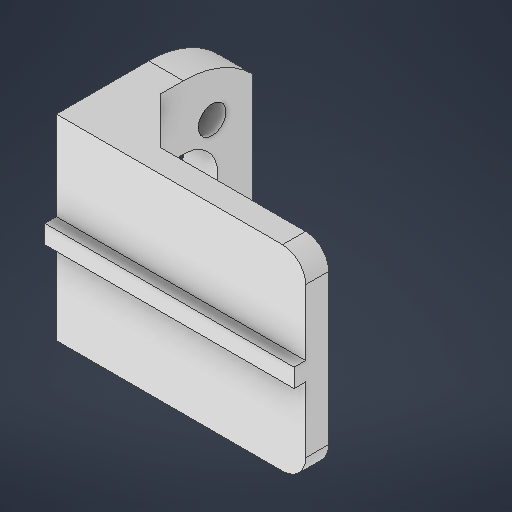
# Autodesk Inventor part: Trzymak2
Saved by Autodesk Inventor 2026 (Build 300175000, 175)
## iProperties
Created: 2025-04-24
Part Number: Trzymak2
Material: Generic
Document SubType Name: Modeling
Designer: isan
Density: 1 g/cm^3
Appearance: Default
Author: isan
Autodesk Inventor part; units mm, degrees
ref_plane "YZ Plane" through (0, 0, 0) normal (1, 0, 0) x (0, 1, 0)
ref_plane "XZ Plane" through (0, 0, 0) normal (0, 1, 0) x (-1, 0, 0)
ref_plane "XY Plane" through (0, 0, 0) normal (0, 0, 1) x (1, 0, 0)
sketch "Sketch1" plane through (0, 0, 0) normal (0, 1, 0) x (-1, 0, 0)
  line L0 (-10.8, 8.5) -> (10.8, 8.5)
  line L1 (10.8, 8.5) -> (10.8, -8.5)
  line L2 (10.8, -8.5) -> (-10.8, -8.5)
  line L3 (-10.8, -8.5) -> (-10.8, 8.5)
  line L4 (-10.8, 8.5) -> (10.8, -8.5) construction
  line L5 (10.8, 8.5) -> (-10.8, -8.5) construction
  point P0 (0, 0)
  dimension "d0" = 21.6
  dimension "d1" = 17
  constraints: 12 end point, 2 midpoint, 2 parallel, 1 horizontal, 1 perpendicular
  measures "d0" distance of L1.end L2.end
  measures "d1" distance of L0.end L1.end
extrude "Extrusion1" add sketch "Sketch1" along normal blind 2
sketch "Sketch2" plane through (0, 2, 0) normal (0, 1, 0) x (1, 0, 0)
  line L0 (-10.8, 8.5) -> (-10.8, -8.5) projected
  line L1 (-10.8, -8.5) -> (-7.8, -8.5)
  line L2 (-7.8, -8.5) -> (-7.8, 8.5)
  line L3 (-7.8, 8.5) -> (-10.8, 8.5)
  line L4 (-10.8, 8.5) -> (-10.8, -8.5)
  point P0 (0, 0)
  point P1 (-10.8, 0)
  point P2 (-10.8, 8.5)
  dimension "d4" = 3
  dimension "d5" = 17
  constraints: 8 end point, 2 midpoint, 2 parallel, 1 horizontal, 1 perpendicular
  measures "d4" distance of L2.end L3.end
  measures "d5" distance of L1.end L2.end
extrude "Extrusion2" add sketch "Sketch2" along normal blind 12
sketch "Sketch3" plane through (-7.8, 2, 8.5) normal (1, 0, 0) x (0, 0, -1)
  circle A0 centre (8.5, 6) radius 3
  line L0 (0, 12) -> (17, 12) projected
  line L1 (17, 0) -> (17, 12) projected
  circle A1 centre (4.1699, 8.5) radius 1.2
  line L2 (0, -2) -> (0, 12) projected
  line L3 (0, 6) -> (17, 6) construction
  line L4 (1.8753, 9.8248) -> (15.1247, 2.1752) construction
  circle A2 centre (12.8301, 3.5) radius 1.2
  point P0 (8.5, -2)
  point P1 (8.5, 6)
  dimension "d8" = 6
  dimension "d9" = 6
  dimension "d10" = 8.5
  dimension "d11" = 2.4
  dimension "d12" = -30
  dimension "d13" = 5
  dimension "d14" = 2.4
  dimension "d15" = 5
  constraints: 4 end point, 3 centre point, 3 midpoint, 3 point on line
  measures "d8" diameter of A0
  measures "d9" distance from line of L0 A0.centre
  measures "d10" distance from line of L1 A0.centre
  measures "d11" diameter of A1
  measures "d12" angle of L3 L4
  measures "d13" distance of A0.centre A1.centre
  measures "d14" diameter of A2
  measures "d15" distance of A0.centre A2.centre
extrude "Extrusion3" cut sketch "Sketch3" against normal blind 5
sketch "Sketch4" plane through (-10.8, 0, -8.5) normal (-1, 0, 0) x (0, 0, 1)
  circle A0 centre (8.5, 8) radius 3 projected
  circle A1 centre (8.5, 8) radius 8.5
  line L0 (0, 0) -> (0, 14) projected
  circle A2 centre (8.5, 8) radius 12.6892
  line L1 (8.5, 8) -> (-4.1892, 8)
  line L2 (8.5, 8) -> (21.1892, 8)
  point P0 (8.5, 0)
  point P1 (17, 8)
  point P2 (0, 8)
  dimension "d18" = 17
  constraints: 4 end point, 2 centre point, 2 coincident, 2 point on circle, 1 horizontal, 1 point on line, 1 tangent
  measures "d18" diameter of A1
extrude "Extrusion4" cut sketch "Sketch4" against normal blind 5 contours A1 L1 A2 L2 picked at (-2.5876, 9.6903)
sketch "Sketch5" plane through (-10.8, 0, -8.5) normal (-1, 0, 0) x (0, 0, 1)
  circle A0 centre (4.1699, 5.5) radius 1.2 projected
  circle A1 centre (12.8301, 10.5) radius 1.2 projected
  line L0 (4.1699, 5.5) -> (12.8301, 10.5) construction
  point P0 (8.5, 0)
  point P1 (8.5, 8)
  constraints: 4 end point, 1 midpoint
extrude "Extrusion6" cut sketch "Sketch5" against normal blind 0.4
sketch "Sketch7" plane through (0, 0, 0) normal (0, -1, 0) x (1, 0, 0)
  line L0 (-10.8, -8.5) -> (-10.8, 8.5) projected
  line L1 (-10.8, 0.8) -> (10.8, 0.8)
  line L2 (10.8, 0.8) -> (10.8, -0.8)
  line L3 (10.8, -0.8) -> (-10.8, -0.8)
  line L4 (-10.8, -0.8) -> (-10.8, 0.8)
  line L5 (10.8, 8.5) -> (10.8, -8.5) projected
  point P0 (0, 0)
  dimension "d27" = 1.6
  dimension "d28" = 0.8
  constraints: 8 end point, 2 parallel, 1 collinear, 1 horizontal, 1 perpendicular, 1 point on line
  measures "d27" distance of L1.end L2.end
  measures "d28" distance from line of point (0, 0) L1
extrude "Extrusion7" add sketch "Sketch7" along normal blind 1
fillet "Fillet1" radius 2 2 edges at (10.8, 1, -8.5) (10.8, 1, 8.5)
sketch "Sketch9" plane through (-7.8, 2, 8.5) normal (1, 0, 0) x (0, 0, -1)
  line L0 (17, 0) -> (16, 0)
  line L1 (16, 0) -> (16, 4)
  line L2 (16, 4) -> (17, 4)
  line L3 (17, 4) -> (17, 0)
  point P0 (8.5, -2)
  dimension "d36" = 1
  dimension "d37" = 4
  constraints: 8 end point, 2 parallel, 1 horizontal, 1 perpendicular
  measures "d36" distance of L1.end L2.end
  measures "d37" distance of L0.end L1.end
extrude "Extrusion9" add sketch "Sketch9" along normal blind 4
chamfer "Chamfer2" distance 4 angle 45 1 edges at (-3.8, 6, -8)
mirror "Mirror2" about plane through (0, 0, 0) normal (0, 0, 1) of "Extrusion9", "Chamfer2"
body "Solid1"
